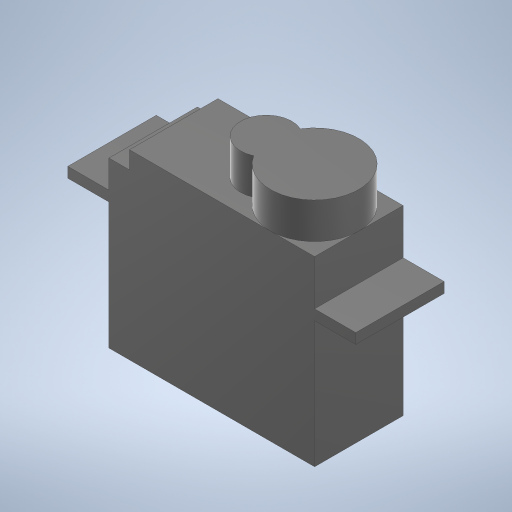
# Autodesk Inventor part: Servo
Saved by Autodesk Inventor 2024.2 (Build 282272000, 272)
## iProperties
Created: 2023-10-03
Part Number: Servo
Material: Generic
Document SubType Name: Modeling
Designer: Alexander Saavedra
Density: 1 g/cm^3
Appearance: Default
Author: Alexander Saavedra
Autodesk Inventor part; units mm, degrees
ref_plane "YZ Plane" through (0, 0, 0) normal (1, 0, 0) x (0, 1, 0)
ref_plane "XZ Plane" through (0, 0, 0) normal (0, 1, 0) x (-1, 0, 0)
ref_plane "XY Plane" through (0, 0, 0) normal (0, 0, 1) x (1, 0, 0)
sketch "Sketch1" plane through (0, 0, 0) normal (0, 0, 1) x (1, 0, 0)
  line L0 (0, 0) -> (-20, 0)
  line L1 (-18, 17.7) -> (0, 17.7)
  line L2 (-20, 17.7) -> (-18, 17.7)
  line L3 (-18, 17.7) -> (-18, 16)
  line L4 (-18, 16) -> (-20, 16)
  line L5 (-20, 16) -> (-20, 13.3)
  line L6 (-20, 13.3) -> (-24, 13.3)
  line L7 (-24, 13.3) -> (-24, 12.3)
  line L8 (-24, 12.3) -> (-20, 12.3)
  line L9 (-20, 0) -> (-20, 12.3)
  line L10 (-20, 13.3) -> (-20, 16)
  line L11 (0, 13.3) -> (4, 13.3)
  line L12 (4, 13.3) -> (4, 12.3)
  line L13 (4, 12.3) -> (0, 12.3)
  line L14 (0, 0) -> (0, 12.3)
  line L15 (0, 13.3) -> (0, 17.7)
  dimension "d0" = 20
  dimension "d1" = 17.7
  dimension "d2" = 2
  dimension "d3" = 1.7
  dimension "d4" = 2.7
  dimension "d5" = 4
  dimension "d6" = 1
  constraints: 32 end point, 7 perpendicular, 2 horizontal, 2 vertical
  measures "d0" distance of L0.start L0.end
  measures "d1" distance of L0.end L2.start
  measures "d2" distance of L1.start L2.start
  measures "d3" distance of L1.start L3.end
  measures "d4" distance of L4.end L5.end
  measures "d5" distance of L5.end L6.end
  measures "d6" distance of L6.end L7.end
extrude "Extrusion1" add sketch "Sketch1" along normal blind 8.6
sketch "Sketch2" plane through (-18, 17.7, 0) normal (0, 1, 0) x (1, 0, 0)
  line L0 (18, 0) -> (0, 0) projected
  line L1 (0, 0) -> (0, -8.6) projected
  line L2 (18, -8.6) -> (0, -8.6) projected
  line L3 (18, 0) -> (18, -8.6) projected
  circle A0 centre (13.7, -4.3) radius 4.3
  constraints: 3 tangent, 1 centre point
extrude "Extrusion2" add sketch "Sketch2" along normal blind 3.5 contours A0
sketch "Sketch3" plane through (-18, 17.7, 8.6) normal (0, 1, 0) x (1, 0, 0)
  line L0 (18, 8.6) -> (18, 4.3) projected
  line L1 (9, 8.6) -> (9, 0)
  line L2 (13.7, 8.6) -> (0, 8.6) projected
  line L3 (13.7, 0) -> (0, 0) projected
  line L4 (6.1752, 8.6) -> (10.4672, 8.6)
  line L5 (6.1752, 0) -> (10.4672, 0)
  circle A0 centre (9, 4.3) radius 2.5
  dimension "d11" = 9
  dimension "d12" = 5
  constraints: 6 end point, 6 point on line, 1 centre point, 1 midpoint, 1 vertical
  measures "d11" distance between parallel lines of L0 L1
  measures "d12" diameter of A0
extrude "Extrusion3" add sketch "Sketch3" along normal up to surface (3.5 mm away)
sketch "Sketch4" plane through (0, 0, 8.6) normal (0, 0, 1) x (1, 0, 0)
  line L0 (-24, 13.3) -> (-24, 12.3) projected
  line L1 (-20, 13.3) -> (-24, 13.3) projected
  line L2 (-20, 16) -> (-20, 13.3) projected
  line L3 (-18, 16) -> (-20, 16) projected
  line L4 (-18, 17.7) -> (-18, 16) projected
  line L5 (-4.3, 17.7) -> (-18, 17.7) projected
  line L6 (0, 17.7) -> (-4.3, 17.7) projected
  line L7 (0, 13.3) -> (0, 17.7) projected
  line L8 (4, 13.3) -> (0, 13.3) projected
  line L9 (4, 12.3) -> (4, 13.3) projected
  line L10 (0, 12.3) -> (4, 12.3) projected
  line L11 (0, 0) -> (0, 12.3) projected
  line L12 (-20, 0) -> (0, 0) projected
  line L13 (-20, 12.3) -> (-20, 0) projected
  line L14 (-24, 12.3) -> (-20, 12.3) projected
sketch "Sketch5" plane through (0, 0, 0) normal (1, 0, 0) x (0, 0, -1)
  line L0 (0, 0) -> (0, 12.3) projected
  line L1 (0, 12.3) -> (-8.6, 12.3) projected
  line L2 (-8.6, 0) -> (-8.6, 12.3) projected
  line L3 (0, 0) -> (-8.6, 0) projected
body "Solid1"
